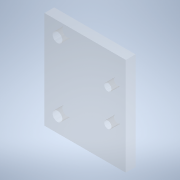
# Autodesk Inventor part: plateencoder
Saved by Autodesk Inventor 2021 (Build 250183000, 183)
## iProperties
Created: 2023-10-29
Part Number: plateencoder
Material: PMMA Plastic
Document SubType Name: Modeling
Designer: M
Density: 1.23642 g/cm^3
Appearance: Polycarbonate - Clear
Mass: 21.6 g
Surface Area: 75.3913 cm^2
Volume: 17.4699 cm^3
Author: M
Autodesk Inventor part; units mm, degrees
ref_plane "YZ Plane" through (0, 0, 0) normal (1, 0, 0) x (0, 1, 0)
ref_plane "XZ Plane" through (0, 0, 0) normal (0, 1, 0) x (-1, 0, 0)
ref_plane "XY Plane" through (0, 0, 0) normal (0, 0, 1) x (1, 0, 0)
sketch "Sketch1" plane through (0, 0, 0) normal (0, 0, 1) x (1, 0, 0)
  line L0 (0, 0) -> (50, 0)
  line L1 (50, 0) -> (50, -60)
  line L2 (50, -60) -> (0, -60)
  line L3 (0, -60) -> (0, 0)
  circle A0 centre (8, -51) radius 3
  circle A1 centre (8, -9) radius 3
  line L4 (8, -51) -> (8, -9)
  circle A2 centre (39, -40) radius 2.25
  circle A3 centre (39, -20) radius 2.25
  line L5 (39, -40) -> (39, -20)
  dimension "d0" = 50
  dimension "d3" = 60
  dimension "d4" = 6
  dimension "d5" = 6
  dimension "d6" = 42
  dimension "d7" = 8
  dimension "d8" = 9
  dimension "d9" = 4.5
  dimension "d10" = 4.5
  dimension "d11" = 20
  dimension "d12" = 11
  dimension "d13" = 20
  constraints: 12 end point, 4 centre point, 2 parallel, 2 vertical, 1 coincident, 1 horizontal, 1 perpendicular
  measures "d0" distance of L1.end L2.end
  measures "d3" distance of L2.end L0.start
  measures "d4" diameter of A0
  measures "d5" diameter of A1
  measures "d6" distance of L4.start L4.end
  measures "d7" distance from line of L3 L4.start
  measures "d8" distance from line of L2 L4.start
  measures "d9" diameter of A2
  measures "d10" diameter of A3
  measures "d11" distance of L5.start L5.end
  measures "d12" distance between parallel lines of L1 L5
  measures "d13" distance from line of L2 L5.start
extrude "Extrusion1" add sketch "Sketch1" along normal blind 6
equation "\"d8\" = -0.5 * d6 + 0.5 * d3"
equation "\"d13\" = -0.5 * d11 + 0.5 * d3"
body "Solid1"
